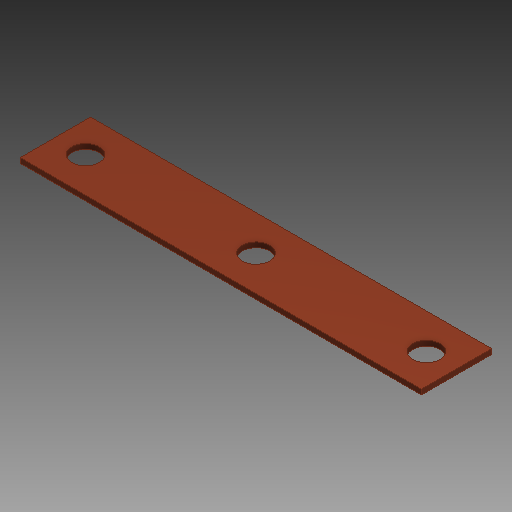
# Autodesk Inventor part: Cu_Cap
Saved by Autodesk Inventor 2019 (Build 230136000, 136)
## iProperties
Created: 2018-05-16
Part Number: Cu_Cap
Material: Copper
Document SubType Name: Modeling
Designer: Phil Erle
Density: 8.94 g/cm^3
Appearance: Copper - Satin
Author: Phil Erle
Autodesk Inventor part; units mm, degrees
ref_plane "YZ Plane" through (0, 0, 0) normal (1, 0, 0) x (0, 1, 0)
ref_plane "XZ Plane" through (0, 0, 0) normal (0, 1, 0) x (-1, 0, 0)
ref_plane "XY Plane" through (0, 0, 0) normal (0, 0, 1) x (1, 0, 0)
sketch "Sketch1" plane through (0, 0, 0) normal (0, 0, 1) x (1, 0, 0)
  line L0 (-40, -7) -> (40, -7)
  line L1 (40, -7) -> (40, 7)
  line L2 (40, 7) -> (-40, 7)
  line L3 (-40, 7) -> (-40, -7)
  line L4 (-40, -7) -> (40, 7) construction
  line L5 (40, -7) -> (-40, 7) construction
  point P0 (0, 0)
  dimension "d0" = 80
  dimension "d1" = 14
  constraints: 12 end point, 2 midpoint, 2 parallel, 1 horizontal, 1 perpendicular
  measures "d0" distance of L2.end L1.end
  measures "d1" distance of L0.end L1.end
extrude "Extrusion1" add sketch "Sketch1" along normal blind 1
sketch "Sketch2" plane through (0, 0, 1) normal (0, 0, 1) x (1, 0, 0)
  point P0 (0, 0)
  point P1 (0, 0)
  constraints: 1 coincident
hole "Hole1" at (0, 0, 1) direction (0, 0, -1) diameter 5.5 depth 8 tip angle 118 clearance for "Countersunk Flat Head Screw DIN EN ISO 2009" size "M5" standard "DIN"
sketch "Sketch3" plane through (0, 0, 1) normal (0, 0, 1) x (1, 0, 0)
  line L0 (-34, 0) -> (34, 0) construction
  point P0 (0, 0)
  point P1 (0, 0)
  dimension "d11" = 68
  constraints: 3 coincident, 2 end point, 1 horizontal, 1 horizontal alignment, 1 midpoint
  measures "d11" distance of L0.start L0.end
hole "Hole2" at (-34, 0, 1) at (34, 0, 1) direction (0, 0, -1) diameter 5.5 depth 8 tip angle 118 clearance for "Countersunk Flat Head Screw DIN EN ISO 2009" size "M5" standard "DIN"
body "Solid1"
